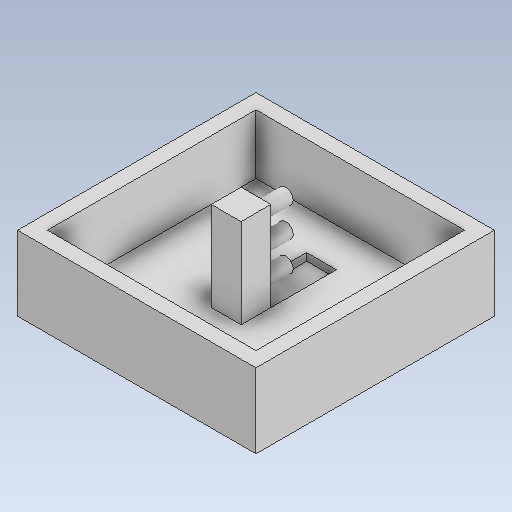
# Autodesk Inventor part: Weight1
Saved by Autodesk Inventor 2020 (Build 240168000, 168)
## iProperties
Created: 2020-04-07
Part Number: Weight1
Material: Generic
Document SubType Name: Modeling
Designer: gman
Density: 1 g/cm^3
Appearance: Default
Mass: 16.6531 g
Surface Area: 113.835 cm^2
Volume: 16.6531 cm^3
Author: gman
Autodesk Inventor part; units mm, degrees
ref_plane "YZ Plane" through (0, 0, 0) normal (1, 0, 0) x (0, 1, 0)
ref_plane "XZ Plane" through (0, 0, 0) normal (0, 1, 0) x (-1, 0, 0)
ref_plane "XY Plane" through (0, 0, 0) normal (0, 0, 1) x (1, 0, 0)
sketch "Sketch1" plane through (0, 0, 0) normal (0, 0, 1) x (1, 0, 0)
  circle A0 centre (0, 6.35) radius 1.5875
  circle A1 centre (0, 0) radius 1.5875
  circle A2 centre (0, -6.35) radius 1.5875
  dimension "d0" = 3.175
  dimension "d1" = 6.35
  dimension "d2" = 6.35
  constraints: 3 centre point, 2 equal radius, 2 vertical alignment, 1 coincident
  measures "d0" diameter of A1
  measures "d1" distance of A2.centre point (0, 0)
  measures "d2" distance of A0.centre point (0, 0)
extrude "Extrusion1" add sketch "Sketch1" along normal blind 6.35
sketch "Sketch2" plane through (0, 6.35, 6.35) normal (0, 0, 1) x (1, 0, 0)
  line L0 (-3.175, 3.175) -> (3.175, 3.175)
  line L1 (3.175, 3.175) -> (3.175, -15.875)
  line L2 (3.175, -15.875) -> (-3.175, -15.875)
  line L3 (-3.175, -15.875) -> (-3.175, 3.175)
  circle A0 centre (0, 0) radius 1.5875 projected
  circle A1 centre (0, -12.7) radius 1.5875 projected
  point P0 (0, -6.35)
  dimension "d5" = 6.35
  dimension "d7" = 3.175
  dimension "d8" = 3.175
  dimension "d11" = 3.175
  constraints: 8 end point, 2 parallel, 1 horizontal, 1 perpendicular
  measures "d5" distance of L0.start L0.end
  measures "d7" distance from line of A0.centre L0
  measures "d8" distance from line of A0.centre L3
  measures "d11" distance from line of A1.centre L2
extrude "Extrusion2" add sketch "Sketch2" along normal blind 6.35 contours L0 L1 L2 L3 | A0 | A1
sketch "Sketch3" plane through (-3.175, -9.525, 6.35) normal (0, -1, 0) x (1, 0, 0)
  line L0 (28.575, 25.4) -> (-22.225, 25.4)
  line L1 (-22.225, 25.4) -> (-22.225, -25.4)
  line L2 (-22.225, -25.4) -> (28.575, -25.4)
  line L3 (28.575, -25.4) -> (28.575, 25.4)
  line L4 (0, 0) -> (6.35, 0) projected
  line L5 (6.35, 0) -> (0, 0)
  line L6 (0, 0) -> (0, -13.97)
  line L7 (0, -13.97) -> (6.35, -13.97)
  line L8 (6.35, -13.97) -> (6.35, 0)
  point P0 (3.175, -6.35)
  dimension "d12" = 50.8
  dimension "d13" = 50.8
  dimension "d14" = 25.4
  dimension "d15" = 25.4
  dimension "d16" = 6.35
  dimension "d17" = 0
  dimension "d18" = 22.225
  dimension "d19" = 13.97
  constraints: 16 end point, 4 parallel, 2 horizontal, 2 perpendicular
  measures "d12" distance of L1.end L2.end
  measures "d13" distance of L0.end L1.end
  measures "d14" distance between parallel lines of L4 L0
  measures "d15" distance from line of point (3.175, -6.35) L1
  measures "d16" distance of L6.end L7.end
  measures "d17" distance between parallel lines of L4 L5
  measures "d18" distance between parallel lines of L1 L6
  measures "d19" distance of L7.end L5.start
extrude "Extrusion3" add sketch "Sketch3" along normal blind 3.175
sketch "Sketch4" plane through (-3.175, -9.525, 6.35) normal (0, 1, 0) x (1, 0, 0)
  line L0 (-22.225, -25.4) -> (-22.225, 25.4) projected
  line L1 (-22.225, 25.4) -> (28.575, 25.4) projected
  line L2 (-22.225, -25.4) -> (28.575, -25.4)
  line L3 (28.575, -25.4) -> (28.575, 25.4)
  line L4 (28.575, 25.4) -> (-22.225, 25.4)
  line L5 (-22.225, 25.4) -> (-22.225, -25.4)
  line L6 (25.4, -22.225) -> (-19.05, -22.225)
  line L7 (-19.05, -22.225) -> (-19.05, 22.225)
  line L8 (-19.05, 22.225) -> (25.4, 22.225)
  line L9 (25.4, 22.225) -> (25.4, -22.225)
  point P0 (3.175, 6.35)
  dimension "d22" = 3.175
  constraints: 16 end point, 4 parallel, 2 perpendicular, 1 horizontal, 3 other
  measures "d22" distance between parallel lines of L2 L6
extrude "Extrusion4" add sketch "Sketch4" along normal blind 12.7
sketch "Sketch5" plane through (-3.175, -12.7, 6.35) normal (0, -1, 0) x (1, 0, 0)
  line L0 (6.35, 0) -> (6.35, -13.97) projected
  line L1 (0, -13.97) -> (0, 0) projected
  line L2 (6.35, 0) -> (0, 0)
  line L3 (0, 0) -> (0, -13.97)
  line L4 (0, -13.97) -> (6.35, -13.97)
  line L5 (6.35, -13.97) -> (6.35, 0)
  point P0 (3.175, -6.35)
  constraints: 8 end point, 2 parallel, 1 horizontal, 1 perpendicular
extrude "Extrusion5" add sketch "Sketch5" against normal blind 1.5875
body "Solid1"
